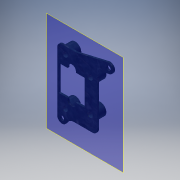
# Autodesk Inventor part: The Holdy Thing
Saved by Autodesk Inventor 2017 (Build 210142000, 142)
## iProperties
Created: 2017-01-05
Part Number: The Holdy Thing
Material: Generic
Document SubType Name: Modeling
Designer: PLTW
Density: 1 g/cm^3
Appearance: Green Polished
Author: PLTW
Autodesk Inventor part; units mm, degrees
ref_plane "YZ Plane" through (0, 0, 0) normal (1, 0, 0) x (0, 1, 0)
ref_plane "XZ Plane" through (0, 0, 0) normal (0, 1, 0) x (-1, 0, 0)
sketch "Sketch1" plane through (0, 0, 0) normal (0, 0, 1) x (1, 0, 0)
  line L0 (-27.8883, 16.9571) -> (-16.5526, 11.23) projected
  arc A0 (-13.2896, 14.9495) -> (-16.5526, 11.23) centre (0, 0) ccw projected
  arc A1 (-8.5326, 14.329) -> (-13.2896, 14.9495) centre (-11.1801, 12.5765) ccw projected
  arc A2 (-8.5326, 14.329) -> (-0.3824, 16.6727) centre (-4.826, 16.7824) ccw projected
  arc A3 (3.3184, 19.7253) -> (-0.3824, 16.6727) centre (2.7917, 16.5943) ccw projected
  arc A4 (7.7895, 18.4234) -> (3.3184, 19.7253) centre (0, 0) ccw projected
  arc A5 (9.2731, 13.8613) -> (7.7895, 18.4234) centre (6.5531, 15.4991) ccw projected
  arc A6 (9.2731, 13.8613) -> (14.8911, 7.5086) centre (13.081, 11.5683) ccw projected
  arc A7 (19.2377, 5.4784) -> (14.8911, 7.5086) centre (16.1841, 4.6088) ccw projected
  arc A8 (19.2377, -5.4784) -> (19.2377, 5.4784) centre (0, 0) ccw projected
  arc A9 (14.8911, -7.5086) -> (19.2377, -5.4784) centre (16.1841, -4.6088) ccw projected
  arc A10 (14.8911, -7.5086) -> (9.2731, -13.8613) centre (13.081, -11.5683) ccw projected
  arc A11 (7.7895, -18.4234) -> (9.2731, -13.8613) centre (6.5531, -15.4991) ccw projected
  arc A12 (3.3184, -19.7253) -> (7.7895, -18.4234) centre (0, 0) ccw projected
  arc A13 (-0.3824, -16.6727) -> (3.3184, -19.7253) centre (2.7917, -16.5943) ccw projected
  arc A14 (-0.3824, -16.6727) -> (-8.5326, -14.329) centre (-4.826, -16.7824) ccw projected
  arc A15 (-13.2896, -14.9495) -> (-8.5326, -14.329) centre (-11.1801, -12.5765) ccw projected
  arc A16 (-18.8605, 6.6618) -> (-13.2896, -14.9495) centre (0, 0) ccw projected
  line L1 (-18.8605, 6.6618) -> (-30.1963, 12.389) projected
  arc A17 (-30.1963, 12.389) -> (-27.8883, 16.9571) centre (0, 0) ccw projected
  circle A18 centre (13.081, -11.5683) radius 1.905 projected
  circle A19 centre (-4.826, -16.7824) radius 1.905 projected
  circle A20 centre (-4.826, 16.7824) radius 1.905 projected
  circle A21 centre (13.081, 11.5683) radius 1.905 projected
  circle A22 centre (-4.826, -16.7824) radius 1.905
  circle A23 centre (-4.826, 16.7824) radius 1.905
  circle A24 centre (13.081, 11.5683) radius 1.905
  circle A25 centre (13.081, -11.5683) radius 1.905
  circle A26 centre (-4.826, -16.7824) radius 4.318 projected
  circle A27 centre (-4.826, 16.7824) radius 4.318 projected
  circle A28 centre (13.081, 11.5683) radius 4.318 projected
  circle A29 centre (13.081, -11.5683) radius 4.318 projected
  circle A30 centre (-4.826, -16.7824) radius 4.318
  circle A31 centre (-4.826, 16.7824) radius 4.318
  circle A32 centre (13.081, 11.5683) radius 4.318
  circle A33 centre (13.081, -11.5683) radius 4.318
  point P0 (0, 0)
  constraints: 8 centre point, 8 coincident, 8 equal radius
ref_plane "Work Plane1" through (-15.5702, -32.385, 7.2898) normal (0, 0, -1) x (0, 1, 0)
extrude "Extrusion1" add sketch "Sketch1" along normal up to surface (7.2898 mm away) contours A26 | A27 | A28 | A29
ref_plane "Work Plane2" through (9.6393, 0, 7.2898) normal (0, 0, -1) x (-1, 0, 0)
sketch "Sketch3" plane through (9.6393, 0, 7.2898) normal (0, 0, -1) x (-1, 0, 0)
  circle A0 centre (16.5735, -23.749) radius 2.159 projected
  line L0 (-24.7015, 32.385) -> (-24.7015, -32.385) projected
  line L1 (-24.7015, -32.385) -> (25.2095, -32.385) projected
  line L2 (25.2095, -32.385) -> (25.2095, 32.385) projected
  line L3 (25.2095, 32.385) -> (-24.7015, 32.385) projected
  line L4 (6.6548, -10.0203) -> (6.6548, -9.271) projected
  line L5 (6.6548, -9.271) -> (0.3683, -9.271) projected
  line L6 (0.3683, -9.271) -> (0.3683, 9.271) projected
  line L7 (0.3683, 9.271) -> (6.6548, 9.271) projected
  line L8 (6.6548, 9.271) -> (6.6548, 10.0203) projected
  arc A1 (12.6238, 10.0203) -> (6.6548, 10.0203) centre (9.6393, 10.0203) ccw projected
  line L9 (12.6238, 10.0203) -> (12.6238, 9.271) projected
  line L10 (12.6238, 9.271) -> (18.9103, 9.271) projected
  line L11 (18.9103, 9.271) -> (18.9103, -9.271) projected
  line L12 (18.9103, -9.271) -> (12.6238, -9.271) projected
  line L13 (12.6238, -9.271) -> (12.6238, -10.0203) projected
  arc A2 (6.6548, -10.0203) -> (12.6238, -10.0203) centre (9.6393, -10.0203) ccw projected
  circle A3 centre (-16.5735, 23.749) radius 2.159 projected
  circle A4 centre (16.5735, -23.749) radius 1.524 projected
  circle A5 centre (-16.5735, 23.749) radius 1.524 projected
  circle A6 centre (-16.5735, 23.749) radius 1.524
  circle A7 centre (16.5735, -23.749) radius 1.524
  point P0 (9.6393, 0)
  constraints: 2 centre point, 2 coincident, 2 concentric
extrude "Extrusion2" add sketch "Sketch3" along normal blind 1.27 contours A0 | A3
ref_plane "Work Plane3" through (9.6393, 0, 7.2898) normal (0, 0, -1) x (-1, 0, 0)
sketch "Sketch4" plane through (9.6393, 0, 7.2898) normal (0, 0, -1) x (-1, 0, 0)
  line L0 (20.0025, 21.8624) -> (6.4823, 21.8624)
  line L1 (-8.5217, 16.7824) -> (-8.5217, -21.8624)
  line L2 (20.0025, -9.6633) -> (20.0025, 21.8624)
  circle A0 centre (16.5735, -23.749) radius 1.524 projected
  line L3 (-8.5217, -21.8624) -> (13.1445, -21.8624)
  circle A1 centre (-16.5735, 23.749) radius 1.524 projected
  circle A2 centre (14.4653, -16.7824) radius 4.318 projected
  circle A3 centre (14.4653, 16.7824) radius 1.905 projected
  circle A4 centre (-3.4417, 11.5683) radius 1.905 projected
  line L4 (-8.5217, 16.7824) -> (-8.5217, 17.1543)
  circle A5 centre (14.4653, 16.7824) radius 1.905 projected
  circle A6 centre (14.4653, 16.7824) radius 4.318 projected
  circle A7 centre (-3.4417, 11.5683) radius 1.905 projected
  circle A8 centre (-3.4417, 11.5683) radius 4.318 projected
  circle A9 centre (-3.4417, -11.5683) radius 1.905 projected
  circle A10 centre (-3.4417, -11.5683) radius 4.318 projected
  line L5 (-8.5217, 18.3405) -> (-8.5217, 17.1543)
  line L6 (16.5735, -23.749) -> (16.5735, -9.6633) construction
  line L7 (13.1445, -23.749) -> (13.1445, -21.8624)
  line L8 (20.0025, -9.6633) -> (20.0025, -23.749)
  arc A11 (13.1445, -23.749) -> (20.0025, -23.749) centre (16.5735, -23.749) ccw
  circle A12 centre (16.5735, -23.749) radius 2.159 projected
  line L9 (-16.5735, 23.749) -> (5.5021, 18.5765) construction
  line L10 (-15.7912, 27.0876) -> (6.2843, 21.9151)
  line L11 (-8.5217, 18.3405) -> (-17.3558, 20.4104)
  arc A13 (-15.7912, 27.0876) -> (-17.3558, 20.4104) centre (-16.5735, 23.749) ccw
  arc A14 (6.4823, 21.8624) -> (6.2843, 21.9151) centre (5.5021, 18.5765) ccw
  circle A15 centre (-16.5735, 23.749) radius 2.159 projected
  circle A16 centre (16.5735, -23.749) radius 2.159 projected
  line L12 (-24.7015, 32.385) -> (-24.7015, -32.385) projected
  line L13 (-24.7015, -32.385) -> (25.2095, -32.385) projected
  line L14 (25.2095, -32.385) -> (25.2095, 32.385) projected
  line L15 (25.2095, 32.385) -> (-24.7015, 32.385) projected
  line L16 (6.6548, -10.0203) -> (6.6548, -9.271) projected
  line L17 (6.6548, -9.271) -> (0.3683, -9.271) projected
  line L18 (0.3683, -9.271) -> (0.3683, 9.271) projected
  line L19 (0.3683, 9.271) -> (6.6548, 9.271) projected
  line L20 (6.6548, 9.271) -> (6.6548, 10.0203) projected
  arc A17 (12.6238, 10.0203) -> (6.6548, 10.0203) centre (9.6393, 10.0203) ccw projected
  line L21 (12.6238, 10.0203) -> (12.6238, 9.271) projected
  line L22 (12.6238, 9.271) -> (18.9103, 9.271) projected
  line L23 (18.9103, 9.271) -> (18.9103, -9.271) projected
  line L24 (18.9103, -9.271) -> (12.6238, -9.271) projected
  line L25 (12.6238, -9.271) -> (12.6238, -10.0203) projected
  arc A18 (6.6548, -10.0203) -> (12.6238, -10.0203) centre (9.6393, -10.0203) ccw projected
  circle A19 centre (-16.5735, 23.749) radius 2.159 projected
  point P0 (9.6393, 0)
  point P1 (16.5735, -16.7062)
  point P2 (-5.5357, 21.1627)
  dimension "d6" = 5.08
  dimension "d7" = 5.08
  dimension "d8" = 5.08
  dimension "d15" = 1.27
  dimension "d16" = 1.27
  constraints: 28 end point, 6 point on circle, 6 tangent, 4 parallel, 3 centre point, 3 vertical, 2 midpoint, 1 coincident, 1 horizontal, 1 perpendicular, 1 point on line
  measures "d6" distance from line of L0 A3.centre
  measures "d7" distance from line of L1 A4.centre
  measures "d8" distance from line of A2.centre L3
  measures "d15" radial gap between concentric circles of A12 A11
  measures "d16" radial gap between concentric circles of A15 A13
extrude "Extrusion3" add sketch "Sketch4" along normal blind 1.27 contours L2 L8 A11 L7 L3 L1 L4 L5 L11 A13 L10 A14 L0
fillet "Fillet1" radius 6.35 3 edges at (18.161, 18.3405, 6.6548) (3.157, 21.8624, 6.6548) (-3.5052, -21.8624, 6.6548)
fillet "Fillet2" radius 3.175 2 edges at (18.161, -21.8624, 6.6548) (-10.3632, 21.8624, 6.6548)
fillet "Fillet3" radius 0.635 4 edges at (-9.144, 16.7824, 6.0198) (8.763, 11.5683, 6.0198) (8.763, -11.5683, 6.0198) (-9.144, -16.7824, 6.0198)
sketch "Sketch5" plane through (13.081, 11.5683, 0) normal (0, 0, -1) x (-1, 0, 0)
  circle A0 centre (0, 0) radius 1.905 projected
  circle A1 centre (0, 0) radius 4.318 projected
  circle A2 centre (17.907, 5.2141) radius 1.905 projected
  circle A3 centre (17.907, -28.3507) radius 1.905 projected
  circle A4 centre (0, -23.1367) radius 1.905 projected
  circle A5 centre (17.907, 5.2141) radius 1.3335
  circle A6 centre (0, 0) radius 1.3335
  circle A7 centre (0, -23.1367) radius 1.3335
  circle A8 centre (17.907, -28.3507) radius 1.3335
  point P0 (13.081, -11.5683)
  dimension "d22" = 2.667
  constraints: 4 centre point, 4 coincident, 3 equal radius
  measures "d22" diameter of A5
extrude "Extrusion4" add sketch "Sketch5" against normal up to surface (7.2898 mm away) contours A0 | A2 | A3 | A4
chamfer "Chamfer1" distance 0.635 angle 45 6 edges at (14.4145, -11.5683, 0) (-3.4925, -16.7824, 0) (-3.4925, 16.7824, 0) (14.4145, 11.5683, 0) (27.7368, 23.749, 6.0198) (-5.4102, -23.749, 6.0198)
equation "\"d7\" = d6"
equation "\"d8\" = d5"
equation "\"d16\" = d15"
equation "\"d5\" = 5.08"
body "Solid1"
